table_rim (Autodesk Fusion 360 design; units mm, degrees)
Autodesk Fusion 360 part; units mm, degrees
sketch "Sketch1" plane through (0, 0, 0) normal (0, 1, 0) x (1, 0, 0)
  line L0 (0, 0) -> (0, -32)
  line L1 (0, -32) -> (15, -32)
  line L2 (15, -32) -> (15, -22)
  line L3 (15, -22) -> (5, -22)
  line L4 (5, -22) -> (5, -5)
  line L5 (5, -5) -> (15, -5)
  line L6 (15, -5) -> (15, 0)
  line L7 (15, 0) -> (0, 0)
  dimension "d1" = 15
  dimension "d2" = 32
  dimension "d3" = 10
  dimension "d4" = 17
  dimension "d5" = 10
  dimension "d7" = 15
  constraint coincident L0.start L7.end
  constraint vertical L0
  constraint perpendicular L0 L1
  constraint perpendicular L1 L2
  constraint perpendicular L2 L3
  constraint perpendicular L1 L4
  constraint perpendicular L4 L5
  constraint perpendicular L5 L6
  constraint perpendicular L0 L7
  measures "d1" distance of L0.end L1.end
  measures "d2" distance of L0.start L0.end
  measures "d3" distance of L1.end L2.end L0.end
  measures "d4" distance of L3.end L4.end L0.end
  measures "d5" distance of L2.end L3.end L0.end
  measures "d7" distance of L6.end L0.start
extrude "Extrude1" add sketch "Sketch1" along normal blind 40
fillet "Fillet1" radius 5 1 edges at (15, 20, 0)
fillet "Fillet2" radius 4 1 edges at (0, 20, 0)
fillet "Fillet3" radius 5 1 edges at (0, 20, 32)
equation "d2 = 17 mm + 10 mm + 5 mm"
